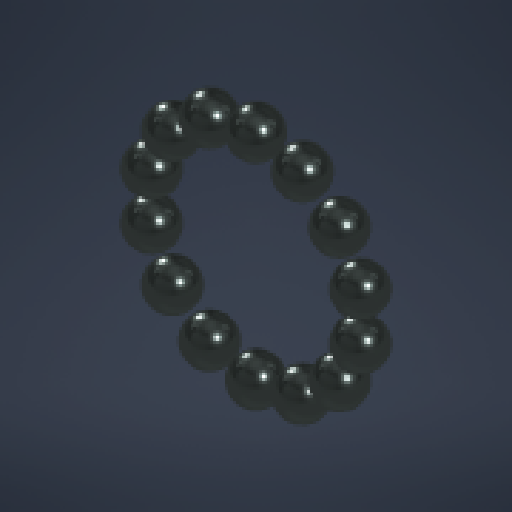
# Autodesk Inventor part: Balls
Saved by Autodesk Inventor 2023.4 (Build 274418000, 418)
## iProperties
Created: 2025-09-28
Part Number: Balls
Material: Generic
Document SubType Name: Modeling
Designer: Malthe Sennels
Density: 1 g/cm^3
Appearance: Gunmetal - Polished
Author: Malthe Sennels
Autodesk Inventor part; units mm, degrees
ref_plane "YZ Plane" through (0, 0, 0) normal (1, 0, 0) x (0, 1, 0)
ref_plane "XZ Plane" through (0, 0, 0) normal (0, 1, 0) x (-1, 0, 0)
ref_plane "XY Plane" through (0, 0, 0) normal (0, 0, 1) x (1, 0, 0)
sketch "Sketch1" plane through (0, 0, 0) normal (0, 0, 1) x (1, 0, 0)
  circle A0 centre (0, 0) radius 8.475
  circle A1 centre (0, 0) radius 13.125 projected
  line L0 (0, 8.475) -> (0, 10.8) construction
  line L1 (0, 0) -> (0, 8.475)
  circle A2 centre (0, 10.8) radius 2.25
  line L2 (0, 8.55) -> (0, 13.05)
  dimension "d0" = 2.325
  dimension "d1" = 4.5
  constraints: 6 end point, 3 vertical, 2 point on circle, 1 centre point, 1 coincident, 1 midpoint, 1 vertical alignment, 2 other
  measures "d0" distance of L0.start L0.end
  measures "d1" diameter of A2
revolve "Revolution1" add sketch "Sketch1" angle 360 about axis through (0, 8.55, 0) along (0, 1, 0) picked at (0.6345, 11.3676) contours A2 L2
pattern_circular "Circular Pattern1" count 14 over 360 about axis through (0, 0, -10) along (0, 0, 1) of "Revolution1"
body "Solid1"
